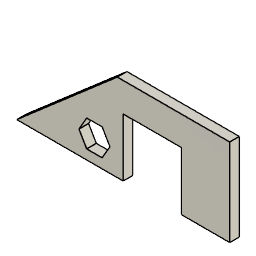
base_pillar (Autodesk Fusion 360 design; units mm, degrees)
part number: 2026-06-29-19-42-22-041
Autodesk Fusion 360 part; units mm, degrees
sketch "Sketch1" plane through (0, 0, 0) normal (0, 1, 0) x (1, 0, 0)
  line L0 (110, 0) -> (41.4831, 0)
  line L1 (51.9615, -45) -> (110, -45)
  line L2 (110, -45) -> (110, 0)
  line L3 (41.4831, 0) -> (0, 0)
  line L4 (0, 0) -> (51.9615, -45)
  dimension "d1" = 110
  dimension "d2" = 45
  dimension "d4" = 58.0385
  constraint horizontal L0
  constraint horizontal L1
  constraint vertical L2
  constraint coincident L3.end L4.start
  measures "d1" distance of L3.end L0.start
  measures "d2" distance of L0.start L1.end
  measures "d4" distance of L1.start L1.end
extrude "Extrude1" add sketch "Sketch1" along normal blind 5
sketch "Sketch2" plane through (0, 0, 0) normal (0, -1, 0) x (1, 0, 0)
  line L0 (51.9615, 45) -> (0, 0)
  line L1 (0, 0) -> (110, 0)
  line L2 (110, 0) -> (110, 45)
  line L3 (110, 45) -> (51.9615, 45)
  line L4 (55, 0) -> (85, 0)
  line L5 (85, 0) -> (85, 30)
  line L6 (85, 30) -> (55, 30)
  line L7 (55, 30) -> (55, 0)
  line L8 (44.1386, 5) -> (48.1184, 11.8931)
  line L9 (48.1184, 11.8931) -> (44.1386, 18.7862)
  line L10 (44.1386, 18.7862) -> (36.1791, 18.7862)
  line L11 (36.1791, 18.7862) -> (32.1994, 11.8931)
  line L12 (32.1994, 11.8931) -> (36.1791, 5)
  line L13 (36.1791, 5) -> (44.1386, 5)
  point P0 (40.1589, 11.8931)
  dimension "d8" = 25
  dimension "d9" = 15
  dimension "d11" = 5
  constraint horizontal L4
  constraint vertical L5
  constraint horizontal L6
  constraint vertical L7
  constraint midpoint L1 L4.start
  measures "d8" distance of L2 L5
  measures "d9" distance of L3 L6
  measures "d11" distance of L1 L13
extrude "Extrude2" cut sketch "Sketch2" against normal through all contours L1 L4 L5 L6 L7
extrude "Extrude3" cut sketch "Sketch2" against normal through all contours L8 L9 L10 L11 L12 L13
